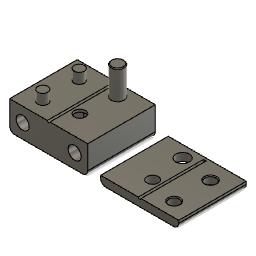
single puller  with rubber band (v4) (Autodesk Fusion 360 archive; units mm, degrees)
design "new pipette holder"
Autodesk Fusion 360 part; units mm, degrees
sketch "Sketch1" plane through (0, 0, 0) normal (0, 1, 0) x (1, 0, 0)
  line L0 (0, 0) -> (30, 0)
  line L1 (30, 0) -> (30, 25)
  line L2 (30, 25) -> (0, 25)
  line L3 (0, 25) -> (0, 0)
  dimension "d1" = 30
  dimension "d2" = 25
  constraint horizontal L0
  constraint vertical L1
  constraint horizontal L2
  constraint vertical L3
  constraint coincident L0.start L3.end
  measures "d1" distance of L0.start L0.end
  measures "d2" distance of L0.start L2.end
extrude "Extrude1" add sketch "Sketch1" along normal blind 11 makes body 1
sketch "Sketch2" plane through (0, 0, 0) normal (0, 0, 1) x (1, 0, 0)
  line L0 (0, 0) -> (30, 0)
  line L1 (30, 0) -> (30, 11)
  line L2 (30, 11) -> (0, 11)
  line L3 (0, 11) -> (0, 0)
  line L4 (0, 11) -> (30, 0) construction
  circle A0 centre (5.001, 5.5) radius 2.5
  line L5 (15, 5.5) -> (15, 11) construction
  circle A1 centre (24.999, 5.5) radius 2.5
  line L6 (5.001, 5.5) -> (2.501, 5.5) construction
  dimension "d5" = 5
  dimension "d59" = 2.501
  constraint coincident L2.end L3.start
  constraint coincident L0.end L1.start
  constraint midpoint L4 L5.start
  constraint midpoint L2 L5.end
  constraint symmetric A0 L5 A1
  constraint coincident A0.centre L6.start
  constraint coincident A0 L6.end
  constraint parallel L2 L6
  measures "d5" diameter of A0
  measures "d59" distance of L3 L6.end
extrude "Extrude2" cut sketch "Sketch2" against normal blind 36 contours A0 bodies 1
sketch "Sketch3" plane through (0, 0, 0) normal (0, 0, 1) x (1, 0, 0)
  circle A0 centre (5.001, 5.5) radius 2.5
  line L0 (0, 0) -> (30, 0)
  line L1 (30, 0) -> (30, 11)
  line L2 (30, 11) -> (0, 11)
  line L3 (0, 11) -> (0, 0)
  circle A1 centre (15, 11) radius 0.5
  dimension "d9" = 1
  constraint midpoint L2 A1.centre
  measures "d9" diameter of A1
extrude "Extrude3" cut sketch "Sketch3" against normal blind 30 contours L2 A1 picked at (14.8961, 10.7714) bodies 1
sketch "Sketch4" plane through (0, 11, 0) normal (0, 1, 0) x (-1, 0, 0)
  line L0 (-15.5, -25) -> (-15.5, 0)
  line L1 (-15.5, 0) -> (-30, 0)
  line L2 (-30, 0) -> (-30, -25)
  line L3 (-30, -25) -> (-15.5, -25)
  line L4 (-15.5, -25) -> (-30, 0) construction
  line L5 (-30, -25) -> (-15.5, 0) construction
  circle A0 centre (-18.5, -8.5) radius 2.15
  dimension "d12" = 4.3
  constraint coincident L0.start L3.end
  constraint coincident L1.end L2.start
  constraint coincident L2.end L3.start
  constraint coincident L0.end L1.start
  measures "d12" diameter of A0
extrude "Extrude4" cut sketch "Sketch4" against normal blind 30 contours A0 bodies 1
sketch "Sketch5" plane through (0, 11, 0) normal (0, 1, 0) x (-1, 0, 0)
  line L0 (-14.5, 0) -> (-14.5, -25)
  line L1 (-14.5, -25) -> (0, -25)
  line L2 (0, -25) -> (0, 0)
  line L3 (0, 0) -> (-14.5, 0)
  line L4 (-10, -12.5) -> (1.5, -12.5) construction
  line L5 (0, -25) -> (-14.5, 0) construction
  line L6 (-7.25, -12.5) -> (-7.25, -26) construction
  circle A0 centre (-7.25, -19.5) radius 1.95
  circle A1 centre (-7.25, -5.5) radius 1.95
  dimension "d15" = 3.9
  constraint perpendicular L2 L4
  constraint coincident L1.end L2.start
  constraint coincident L0.start L3.end
  constraint midpoint L5 L6.start
  constraint perpendicular L1 L6
  constraint coincident L6 A0.centre
  constraint symmetric L4 A0 A1
  measures "d15" diameter of A0
extrude "Extrude5" add sketch "Sketch5" along normal blind 4 contours A0 | A1 bodies 1
sketch "Sketch7" plane through (0, 11, 0) normal (0, 1, 0) x (-1, 0, 0)
  circle A0 centre (-18.5, -8.5) radius 2.15
  line L0 (-15.5, -25) -> (-15.5, 0)
  line L1 (-15.5, 0) -> (-30, 0)
  line L2 (-30, 0) -> (-30, -25)
  line L3 (-30, -25) -> (-15.5, -25)
  line L4 (-9, -19.5) -> (-33.5, -19.5) construction
  circle A1 centre (-20, -21.5) radius 2.5
  constraint perpendicular L2 L4
extrude "Extrude7" add sketch "Sketch7" along normal blind 11 contours A1 bodies 1
fillet "Fillet2" radius 0.3 1 edges at (22.3308, 22, -22.404) on bodies 1
sketch "Sketch8" plane through (0, 0, 0) normal (0, -1, 0) x (1, 0, 0)
  circle A0 centre (18.5, -8.5) radius 2.15
  line L0 (0, 0) -> (0, -25)
  line L1 (0, -25) -> (30, -25)
  line L2 (30, -25) -> (30, 0)
  line L3 (30, 0) -> (0, 0)
  line L4 (22.65, -8.5) -> (20.575, -4.906)
  line L5 (20.575, -4.906) -> (16.425, -4.906)
  line L6 (16.425, -4.906) -> (14.35, -8.5)
  line L7 (14.35, -8.5) -> (16.425, -12.094)
  line L8 (16.425, -12.094) -> (20.575, -12.094)
  line L9 (20.575, -12.094) -> (22.65, -8.5)
  point P0 (18.5, -8.5)
  dimension "d27" = 4.15
  constraint coincident P0 A0.centre
  measures "d27" distance of L4.start P0
extrude "Extrude8" cut sketch "Sketch8" against normal blind 10 contours L4 L5 L6 L7 L8 L9 bodies 1
ref_plane "WorkPlane1" through (7.25, 29, -12.5) normal (0, 1, 0) x (0, 0, 1) in component "top bit"
sketch "Sketch1 (2)" plane through (0, 29, 0) normal (0, 1, 0) x (1, 0, 0) in component "top bit"
  line L0 (0, 25) -> (30, 25)
  line L1 (30, 25) -> (30, 0)
  line L2 (30, 0) -> (0, 0)
  line L3 (0, 0) -> (0, 25)
  constraint horizontal L0
  constraint vertical L1
  constraint horizontal L2
  constraint vertical L3
extrude "Extrude1'" add sketch "Sketch1 (2)" along normal blind 3 separate body makes body 2 in component "top bit"
sketch "Sketch2 (2)" plane through (0, 32, 0) normal (0, 1, 0) x (-1, 0, 0) in component "top bit"
  line L0 (0, 0) -> (-30, 0)
  line L1 (-30, 0) -> (-30, -25)
  line L2 (-30, -25) -> (0, -25)
  line L3 (0, -25) -> (0, 0)
  circle A0 centre (-7.25, -5.5) radius 2
  circle A1 centre (-20, -21.5) radius 2.5
  circle A2 centre (-18.5, -8.5) radius 2.15
  circle A3 centre (-7.25, -5.5) radius 2.1
  line L4 (0, -25) -> (-30, 0) construction
  line L5 (-30, -25) -> (-15, -12.5) construction
  line L6 (-15, -12.5) -> (0, -12.5) construction
  circle A4 centre (-7.25, -19.5) radius 2.1
  circle A5 centre (-20, -21.5) radius 2.6125
  dimension "d33" = 4.2
  dimension "d38" = 5.225
  constraint concentric A0 A3
  constraint coincident L2.end L3.start
  constraint coincident L0.end L1.start
  constraint coincident L1.end L2.start
  constraint midpoint L4 L5.end
  constraint midpoint L3 L6.end
  constraint symmetric A3 L6 A4
  constraint concentric A1 A5
  measures "d33" diameter of A3
  measures "d38" diameter of A5
extrude "Extrude2'" cut sketch "Sketch2 (2)" against normal blind 5 contours A0 | A4 bodies 2 in component "top bit"
fillet "Fillet1" radius 0.3 2 edges at (9.1147, 29, -6.2232) (9.2079, 29, -20.2594) on bodies 2 in component "top bit"
extrude "Extrude3'" cut sketch "Sketch2 (2)" against normal blind 5 contours A1 | A5 bodies 2 in component "top bit"
extrude "Extrude4'" cut sketch "Sketch2 (2)" against normal blind 9 contours A2 bodies 2 in component "top bit"
sketch "Sketch3 (2)" plane through (0, 0, 0) normal (0, 0, 1) x (1, 0, 0) in component "top bit"
  line L0 (0, 29) -> (30, 29)
  line L1 (30, 29) -> (30, 32)
  line L2 (30, 32) -> (0, 32)
  line L3 (0, 32) -> (0, 29)
  line L4 (15, 11) -> (15, 37.4734) construction
  circle A0 centre (15, 29) radius 0.5
  dimension "d43" = 1
  constraint perpendicular L2 L4
  constraint midpoint L0 A0.centre
  measures "d43" diameter of A0
extrude "Extrude5'" cut sketch "Sketch3 (2)" against normal blind 100 contours L0 A0 picked at (15.1222, 29.2116) bodies 2 in component "top bit"
move_body "Move1" bodies 2 to x (1, 0, 0) y (0, 1, 0) z (0, 0, 1) at (0, -18, 0) in component "top bit"
move_body "Move2" bodies 2 to x (-1, 0, 0) y (0, -1, 0) z (0, 0, 1) at (64.9701, 14, 0) in component "top bit"
fillet "Fillet3" radius 2 2 edges at (30, 0, -12.5) (0, 0, -12.5) on bodies 1
fillet "Fillet2'" radius 2 2 edges at (34.9701, 0, -12.5) (64.9701, 0, -12.5) on bodies 2 in component "top bit"
extrude "Extrude9" add 1 faces at (24.4835, 7.261, -25) along direction (0, 0, -1) blind 1 on bodies 1 bodies 1
sketch "Sketch9" plane through (0, 0, -26) normal (0, 0, -1) x (-1, 0, 0)
  arc A0 (-2, 0) -> (0, 2) centre (-2, 2) ccw
  line L0 (0, 2) -> (0, 11)
  line L1 (0, 11) -> (-14.5, 11)
  arc A1 (-15.5, 11) -> (-14.5, 11) centre (-15, 11) ccw
  line L2 (-15.5, 11) -> (-30, 11)
  line L3 (-30, 11) -> (-30, 2)
  arc A2 (-30, 2) -> (-28, 0) centre (-28, 2) ccw
  line L4 (-28, 0) -> (-2, 0)
  circle A3 centre (-5.001, 5.5) radius 2.5
  arc A4 (-15.5, 11) -> (-14.5, 11) centre (-15, 11) ccw
  line L5 (-15.5, 11) -> (-14.5, 11)
  constraint concentric A1 A4
  constraint coincident A1.start L2.start
  constraint coincident L1.end A1.end
extrude "Extrude10" add sketch "Sketch9" against normal blind 1 contours A1 A4 L5 bodies 1
extrude "Extrude6" add 1 faces at (40.4701, 2, -25) along direction (0, 0, -1) blind 1 on bodies 2 bodies 2 in component "top bit"
sketch "Sketch10" plane through (0, 0, -26) normal (0, 0, -1) x (-1, 0, 0)
  arc A0 (-64.9701, 2) -> (-62.9701, 0) centre (-62.9701, 2) ccw
  line L0 (-62.9701, 0) -> (-36.9701, 0)
  arc A1 (-36.9701, 0) -> (-34.9701, 2) centre (-36.9701, 2) ccw
  line L1 (-34.9701, 2) -> (-34.9701, 3)
  line L2 (-34.9701, 3) -> (-49.4701, 3)
  arc A2 (-50.4701, 3) -> (-49.4701, 3) centre (-49.9701, 3) ccw
  line L3 (-50.4701, 3) -> (-64.9701, 3)
  line L4 (-64.9701, 3) -> (-64.9701, 2)
  arc A3 (-50.4701, 3) -> (-49.4701, 3) centre (-49.9701, 3) ccw
  line L5 (-50.4701, 3) -> (-50.4, 3)
  line L6 (-50.4, 3) -> (-49.4701, 3)
  constraint concentric A2 A3
  constraint coincident A2.start L3.start
  constraint parallel L3 L5
  constraint coincident L2.end A2.end
  constraint parallel L2 L6
extrude "Extrude7'" add sketch "Sketch10" against normal blind 1 contours A2 A3 L5 L6 bodies 2 in component "top bit"
extrude "Extrude11" cut sketch "Sketch2" against normal blind 60 contours A1 bodies 1
component "top bit" placed x (1, 0, 0) y (0, 1, 0) z (0, 0, 1) at (0, 0, 0)
